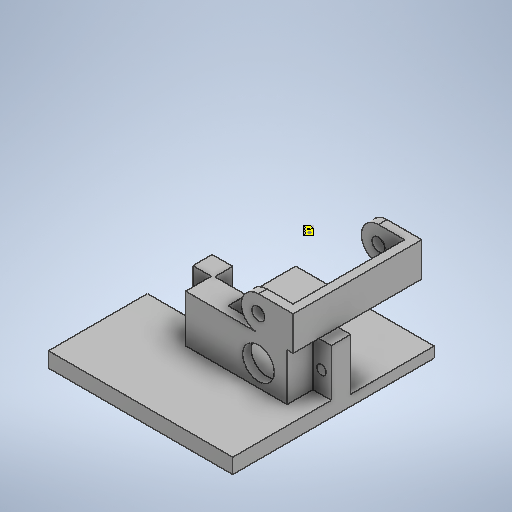
# Autodesk Inventor part: housing_shaft_link_base
Saved by Autodesk Inventor 2025 (Build 290162000, 162)
## iProperties
Created: 2025-09-17
Part Number: housing_shaft_link_base
Material: 一般
Document SubType Name: Modeling
Designer: sooo1
Density: 1 g/cm^3
Appearance: 滑らか - 標準の灰色
Author: sooo1
Autodesk Inventor part; units mm, degrees
sketch "スケッチ1" plane through (0, 0, 0) normal (0, 0, 1) x (1, 0, 0)
  circle A0 centre (0, 0) radius 1.5
  circle A1 centre (0, 0) radius 4
  line L0 (6.1, 4) -> (6.1, -4)
  line L1 (-27.76, 0) -> (17.46, 0) construction
  line L2 (6.1, 4) -> (0, 4)
  line L3 (6.1, -4) -> (0, -4)
  line L4 (6.1, -4) -> (8.1, -4)
  line L5 (8.1, -4) -> (8.1, 4)
  line L6 (8.1, 4) -> (6.1, 4)
  line L7 (0, -13.6) -> (0, 18.6) construction
  circle A2 centre (0, 10) radius 1.5
  circle A3 centre (0, 10) radius 4
  line L8 (6.1, 14) -> (6.1, 6)
  line L9 (6.1, 14) -> (0, 14)
  line L10 (6.1, 6) -> (0, 6)
  line L11 (6.1, 6) -> (8.1, 6)
  line L12 (8.1, 6) -> (8.1, 14)
  line L13 (8.1, 14) -> (6.1, 14)
  line L14 (-16.4, 6.05) -> (6.1, 6.05) construction
  line L15 (6.1, 6.05) -> (6.1, -6.05)
  line L16 (6.1, -6.05) -> (-16.4, -6.05) construction
  line L17 (-16.4, -6.05) -> (-16.4, 6.05)
  line L18 (-16.4, 6.05) -> (6.1, -6.05) construction
  line L19 (6.1, 6.05) -> (-16.4, -6.05) construction
  line L20 (-21.3, 6.05) -> (11, 6.05) construction
  line L21 (11, 6.05) -> (11, -6.05) construction
  line L22 (11, -6.05) -> (-21.3, -6.05)
  line L23 (-21.3, -6.05) -> (-21.3, 6.05) construction
  line L24 (-21.3, 6.05) -> (11, -6.05) construction
  line L25 (11, 6.05) -> (-21.3, -6.05) construction
  line L26 (-21.3, 0) -> (11, 0) construction
  circle A4 centre (-19, 0) radius 1.1
  line L27 (-5.15, 6.05) -> (-5.15, -6.05) construction
  circle A5 centre (0, 0) radius 2.425
  circle A6 centre (0, 0) radius 6.05
  circle A7 centre (0, 0) radius 9
  line L28 (8.1, -7) -> (-21.3, -7)
  line L29 (-21.3, -7) -> (-21.3, 6.05)
  line L30 (-21.3, 6.05) -> (8.1, 6.05)
  line L31 (8.1, 6.05) -> (8.1, -7)
  line L32 (-21.3, -5) -> (-20.943492, -5)
  line L33 (-20.943492, -5) -> (8.1, -5)
  circle A8 centre (8.7, 0) radius 1.1
  line L34 (8.1, 6.05) -> (11, 6.05)
  line L35 (11, 6.05) -> (11, -6.05)
  point P0 (6.1, 0)
  point P1 (6.1, 10)
  point P2 (-5.15, 0)
  point P3 (-5.15, 0)
  point P4 (-0.630476, 6.05)
  point P5 (8.1, 6.05)
  point P6 (8.1, -6.05)
  point P7 (0, 6.05)
  point P8 (-6.663145, 6.05)
  point P9 (-6.663145, -6.05)
  point P10 (0, -6.05)
  point P11 (6.1, 6.617401)
  point P12 (6.663145, 6.05)
  point P13 (0.630476, 6.05)
  point P14 (0.489992, 6.030125)
  point P15 (0.776209, 6)
  point P16 (8.062258, 4)
  point P17 (8.1, 3.923009)
  point P18 (8.062258, -4)
  point P19 (8.1, -3.923009)
  point P20 (6.708204, 6)
  dimension "d0" = 3
  dimension "d1" = 8
  dimension "d3" = 8
  dimension "d4" = 2
  dimension "d11" = 10
  dimension "d21" = 12.1
  dimension "d22" = 22.5
  dimension "d23" = 32.3
  dimension "d24" = 2.2
  dimension "d26" = 27.7
  dimension "d28" = 18
  dimension "d29" = 12.1
  dimension "d30" = 4.85
  dimension "d31" = 6.1
  dimension "d32" = 7
  dimension "d55" = 2
  constraints: 68 end point, 10 midpoint, 9 centre point, 7 collinear, 7 parallel, 6 coincident, 6 horizontal, 6 perpendicular, 5 point on line, 4 point on circle, 2 vertical, 1 concentric, 1 symmetric about line, 19 other
  measures "d0" diameter of A0
  measures "d1" diameter of A1
  measures "d3" distance of L0.start L0.end
  measures "d4" distance between parallel lines of L0 L5
  measures "d11" distance of point (0, 0) point (0, 10)
  measures "d21" distance of L14.end L15.end
  measures "d22" distance of L14.start L14.end
  measures "d23" distance of L20.start L20.end
  measures "d24" diameter of A4
  measures "d26" diameter of A4.centre L27
  measures "d28" diameter of A7
  measures "d29" diameter of A6
  measures "d30" diameter of A5
  measures "d31" distance from line of L15 A5.centre
  measures "d32" distance from line of L28 point (0, 0)
  measures "d55" distance between parallel lines of L28 L33
extrude "押し出し1" add sketch "スケッチ1" along normal blind 2 contours A1 | A1 L2 A6 L3 | L2 L0 L3 A6 | L6 A7 L5 A8 L4 L0 | L6 L5 A7 | A7 L5 L4 | L5 A8 | A5
extrude "押し出し2" add sketch "スケッチ1" against normal blind 7 contours L6 A7 L5 A8 L4 L0 | L6 L5 A7 | A7 L5 L4 | L5 A8
extrude "押し出し3" add sketch "スケッチ1" against normal blind 2 from surface at -7 contours A6 A3 L30 L8 L10 | L10 A3 A6 | L8 L30 A7 L11 | A3 A6 | A6 L30 A3 | A7 L30 L12 L11 | L30 A3 A7 L8 | L8 A7 L30 | A3 L30 A6 | L30 A3 A7 A2 | A7 L8 L13 L12 L30 | A7 A3 L9 L8 | A7 A2 A3
pattern_linear "矩形状パターン1" count 2 spacing 28 along (0, 0, -1) of "押し出し3"
ref_plane "作業平面1" through (0, 0, -17.5) normal (0, 0, 1) x (1, 0, 0)
extrude "押し出し4" add sketch "スケッチ1" against normal up to surface (10.5 mm away) from surface at -7 contours A0 | A1 | A1 L2 A6 L3 | A1 L3 A6 L33 A3 L10 L2 | A6 L10 L15 L2 | L2 L0 L3 A6 | L3 L15 L33 A6 | L6 A7 L5 A8 L4 L0 | L15 L11 A7 L6 | A6 A3 L30 L8 L10 | L10 A3 A6 | L4 A7 L33 L15 | L33 L15 L22 A6 | A6 L33 | A7 L11 L31 L6 | L6 L5 A7 | L8 L30 A7 L11 | A3 A6 | A6 L30 A3 | A7 L5 L4 | L4 L31 L33 A7 | L33 A7 L22 L15 | L22 A7 L28 | L22 A7 L33 A6 | L33 A7 L30 A3 A6 | A7 L30 L12 L11 | A3 L30 A6 | L33 L31 L22 A7 | A7 L28 L29 L22 | L22 L17 L33 A7 | L33 L17 L30 A7 | L5 A8 | L22 L31 L28 A7 | L22 L29 L32 L33 L17 | L33 L32 L29 L30 L17 | A4 | A5
ref_plane "作業平面2" through (0, 0, -13.3) normal (0, 0, 1) x (1, 0, 0)
extrude "押し出し6" cut sketch "スケッチ1" against normal blind 23.4 from surface at -13.3 contours A0 | A1 | A1 L2 A6 L3 | A1 L3 A6 L33 A3 L10 L2 | A6 L10 L15 L2 | L2 L0 L3 A6 | L3 L15 L33 A6 | A6 A3 L30 L8 L10 | L10 A3 A6 | L33 L15 L22 A6 | A6 L33 | A3 A6 | A6 L30 A3 | L22 A7 L33 A6 | L33 A7 L30 A3 A6 | A3 L30 A6 | L22 L17 L33 A7 | L33 L17 L30 A7 | A5
ref_plane "作業平面3" through (0, 0, -9) normal (0, 0, 1) x (1, 0, 0)
extrude "押し出し7" cut sketch "スケッチ1" against normal up to surface (4.3 mm away) from surface at -9 contours A0 | A1 | A1 L2 A6 L3 | A1 L3 A6 L33 A3 L10 L2 | L10 A3 A6 | A6 L33 | A3 A6 | L22 A7 L33 A6 | L33 A7 L30 A3 A6 | A3 L30 A6 | A5 picked at (-0.459231, 6.046871)
extrude "押し出し8" cut sketch "スケッチ1" against normal up to surface (9 mm away) contours A0 | A5
extrude "押し出し9" cut sketch "スケッチ1" against normal through all contours A4
extrude "押し出し10" add sketch "スケッチ1" against normal up to surface (28 mm away) from surface at -9 contours L22 A7 L28 | L8 A7 L30 | A7 L28 L29 L22 | A7 L8 L13 L12 L30 | L22 L31 L28 A7
extrude "押し出し11" cut sketch "スケッチ1" against normal up to surface (19.5 mm away) from surface at -17.5 contours A6 A3 L30 L8 L10 | L10 A3 A6 | L8 L30 A7 L11 | A3 A6 | A6 L30 A3 | A7 L30 L12 L11 | A3 L30 A6
sketch "スケッチ3" plane through (0, 4, 2) normal (0, 1, 0) x (1, 0, 0)
  line L0 (8.1, 0) -> (0, 0) projected
  line L1 (8.1, 9) -> (8.1, 0) projected
  line L2 (6.1, 9) -> (8.1, 9) projected
  line L3 (6.1, 2) -> (6.1, 9) projected
  line L4 (6.1, 2) -> (0, 2) projected
  line L5 (0, 2) -> (0, 0) projected
  line L6 (0, 2) -> (0, 2) projected
  line L7 (0, 2) -> (0, 0) projected
  line L8 (0, 0) -> (0, 0) projected
  line L9 (0, 2) -> (0, 0) projected
  line L10 (-4, 2) -> (-4, 0) projected
  line L11 (-4, 2) -> (0, 2) projected
  line L12 (-4, 0) -> (0, 0) projected
extrude "押し出し12" cut sketch "スケッチ3" against normal through all
extrude "押し出し13" add sketch "スケッチ1" along normal blind 10 and the other way blind 7 contours L33 L15 L22 A6 | A6 L33 | L33 A7 L22 L15 | L22 A7 L28 | L22 A7 L33 A6 | L33 L31 L22 A7 | A7 L28 L29 L22 | L22 L17 L33 A7 | L22 L31 L28 A7 | L22 L29 L32 L33 L17
sketch "スケッチ4" plane through (-21.3, 6.05, -17.5) normal (-1, 0, 0) x (0, 0, 1)
  line L0 (27.5, -13.05) -> (-19.5, -13.05) projected
  line L1 (27.5, -11.05) -> (27.5, -13.05) projected
  line L2 (10.5, -11.05) -> (27.5, -11.05) projected
  line L3 (10.5, 0) -> (10.5, -11.05) projected
  line L4 (10.5, 0) -> (0, 0) projected
  line L5 (0, -12.1) -> (0, 0) projected
  line L6 (0, -12.1) -> (-19.5, -12.1) projected
  line L7 (-19.5, -12.1) -> (-19.5, -13.05) projected
  line L8 (10.5, -11.05) -> (10.5, -13.05)
  point P0 (17.5, -6.05)
  constraints: 2 end point, 1 perpendicular, 1 point on line
extrude "押し出し14" add sketch "スケッチ4" along normal blind 10.7 contours L0 L8 L2 L1
sketch "スケッチ5" plane through (-21.3, -5, -47) normal (0, -1, 0) x (1, 0, 0)
  line L0 (29.4, 10) -> (29.4, 57) projected
  line L1 (29.4, 57) -> (-10.7, 57) projected
  line L2 (-10.7, 40) -> (-10.7, 57) projected
  line L3 (0, 40) -> (-10.7, 40) projected
  line L4 (0, 40) -> (0, 10) projected
  line L5 (0, 10) -> (29.4, 10) projected
  line L6 (-10.7, 43.5) -> (29.4, 43.5) construction
  line L7 (1.2, 51.1) -> (16.4, 51.1)
  line L8 (16.4, 51.1) -> (16.4, 35.9)
  line L9 (16.4, 35.9) -> (1.2, 35.9)
  line L10 (1.2, 35.9) -> (1.2, 51.1)
  line L11 (1.2, 51.1) -> (16.4, 35.9) construction
  line L12 (16.4, 51.1) -> (1.2, 35.9) construction
  line L13 (-10.7, 57) -> (-10.7, 40) projected
  line L14 (-10.7, 40) -> (-10.7, 33.9)
  line L15 (-10.7, 33.9) -> (0, 33.9)
  line L16 (29.4, 57) -> (-10.7, 57) projected
  point P0 (21.3, 47)
  point P1 (8.8, 43.5)
  dimension "d63" = 15.2
  dimension "d64" = 15.2
  dimension "d68" = 13.5
  dimension "d69" = 2
  dimension "d105" = 19.5
  constraints: 18 end point, 4 point on line, 3 perpendicular, 2 midpoint, 2 parallel, 1 horizontal, 1 vertical
  measures "d63" distance of L7.start L7.end
  measures "d64" distance of L9.end L7.start
  measures "d68" distance from line of point (8.8, 43.5) L1
  measures "d69" distance between parallel lines of L15 L9
  measures "d105" distance from line of L13 point (8.8, 43.5)
extrude "押し出し17" add sketch "スケッチ5" along normal blind 1.5 from surface at 2 contours L5 L4 L3 L2 L1 L0 | L7 L8 L9 L10
extrude "押し出し15" cut sketch "スケッチ5" against normal blind 2 from surface at 3.5 contours L7 L8 L9 L10
ref_plane "作業平面4" through (-12.5, -8.5, -11.1) normal (-1, 0, 0) x (0, 0, 1)
ref_plane "作業平面5" through (-20.1, -6.5, -3.5) normal (0, 0, 1) x (1, 0, 0)
extrude "押し出し16" add sketch "スケッチ5" along normal up to surface (3.5 mm away) contours L15 L14 L3 L4
extrude "押し出し18" add sketch "スケッチ1" against normal up to surface (10.5 mm away) from surface at -7 contours L6 A7 L5 A8 L4 L0 | L15 L11 A7 L6 | L4 A7 L33 L15 | A7 L11 L31 L6 | L4 L31 L33 A7 | L33 A7 L22 L15 | L31 L12 L34 L35 L22 L5 A7 A8 | A7 A8 L5 | A7 L30 L12 L11 | L33 L31 L22 A7 | L5 A8 A7 | A8 A7 L5 | L5 A8 | A8 A7
extrude "押し出し19" cut sketch "スケッチ1" against normal through all contours A8 A7 L5 | L5 A8 | A8 A7 picked at (8.4, 0)
sketch "スケッチ6" plane through (8.1, -5, 10) normal (1, 0, 0) x (0, 0, -1)
  line L0 (27.5, -1.05) -> (17, -1.05) projected
  line L1 (17, -1.05) -> (17, 0) projected
  line L2 (17, 0) -> (0, 0) projected
  line L3 (0, 0) -> (0, -3.5) projected
  line L4 (0, -3.5) -> (47, -3.5) projected
  line L5 (47, -1.05) -> (47, -3.5) projected
  line L6 (27.5, -1.05) -> (47, -1.05) projected
  point P0 (10, 5)
extrude "押し出し20" add sketch "スケッチ6" along normal up to surface (2.9 mm away)
sketch "スケッチ7" plane through (6.1, -6.05, -17.5) normal (0, 0, -1) x (-1, 0, 0)
  circle A0 centre (-2.6, 6.05) radius 1.1
  line L0 (-4.9, 0) -> (0, 0)
  line L1 (0, 0) -> (0, 12.1)
  line L2 (0, 12.1) -> (-2, 12.1)
  line L3 (-2, 12.1) -> (-4.9, 12.1)
  line L4 (-4.9, 12.1) -> (-4.9, 0)
  line L5 (0, 12.1) -> (0, 0)
  line L6 (0, 0) -> (6.1, 0)
  arc A1 (6.1, 12.1) -> (6.1, 0) centre (6.1, 6.05) ccw
  line L7 (0, 12.1) -> (6.1, 12.1)
  arc A2 (12.763145, 0) -> (12.763145, 12.1) centre (6.1, 6.05) ccw
  line L8 (12.763145, 0) -> (22.5, 0)
  line L9 (22.5, 0) -> (22.5, 12.1)
  line L10 (12.763145, 12.1) -> (22.5, 12.1)
  line L11 (22.5, 12.1) -> (22.5, 0)
  line L12 (22.5, 0) -> (27.4, 0)
  line L13 (27.4, 0) -> (27.4, 12.1)
  line L14 (27.4, 12.1) -> (22.5, 12.1)
  circle A3 centre (25.1, 6.05) radius 1.1
  line L15 (6.730476, 12.1) -> (12.763145, 12.1)
  line L16 (6.1, 0) -> (12.763145, 0)
  circle A4 centre (6.1, 6.05) radius 2.425
  line L17 (0, 12.1) -> (6.1, 12.1)
  line L18 (6.1, 12.1) -> (6.730476, 12.1)
  line L19 (-0.1, 12.1) -> (-0.1, 0)
  line L20 (-4.9, 0) -> (0, 0)
  line L21 (22.6, 12.1) -> (22.6, 0)
  line L22 (22.5, 0) -> (27.4, 0)
  arc A5 (6.1, 12.2) -> (6.1, -0.1) centre (6.1, 6.05) ccw
  arc A6 (12.83718, -0.067222) -> (12.83718, 12.167222) centre (6.1, 6.05) ccw
  circle A7 centre (6.1, 6.05) radius 3.7
  line L23 (15.2, 12.1) -> (15.2, 0)
  line L24 (27.4, 1.05) -> (-4.9, 1.05)
  line L25 (23.1, 1.05) -> (23.1, 12.1)
  line L26 (-0.6, 1.05) -> (-0.6, 12.1)
  line L27 (22.5, 12.1) -> (22.5, 0)
  line L28 (22.5, 0) -> (27.4, 0)
  line L29 (27.4, 0) -> (27.4, 12.1)
  line L30 (27.4, 12.1) -> (22.5, 12.1)
  point P0 (22.6, 0)
  point P1 (-0.1, 0)
  point P2 (12.89761, 0)
  point P3 (12.89761, 12.1)
  point P4 (4.995464, 12.1)
  point P5 (4.995464, 0)
  point P6 (15.2, 6.05)
  dimension "d80" = 0.1
  dimension "d81" = 0.1
  dimension "d84" = 0.1
  dimension "d85" = 0.1
  dimension "d99" = 2
  dimension "d101" = 2
  dimension "d104" = 7.4
  constraints: 12 end point, 10 point on line, 4 perpendicular, 4 point on circle, 3 centre point, 1 collinear, 1 tangent, 1 vertical
  measures "d80" distance between parallel lines of L19 L1
  measures "d81" distance between parallel lines of L9 L21
  measures "d84" radial gap between concentric circles of A1 A5
  measures "d85" radial gap between concentric circles of A2 A6
  measures "d99" distance from line of L25 A3.centre
  measures "d101" distance from line of L26 A0.centre
  measures "d104" diameter of A7
extrude "押し出し21" cut sketch "スケッチ7" against normal up to surface (4.2 mm away) contours L19 L24 L1 L0 | L19 L2 L1 A5 L24 | A5 L1 | L9 L24 L21 L12 | L9 L14 L21 L24
sketch "スケッチ7 outline for 押し出し22" plane through (6.1, -6.05, -17.5) normal (0, 0, -1) x (-1, 0, 0)
  arc A0 (12.763145, 12.1) -> (12.763145, 0) centre (6.1, 6.05) cw
  line L0 (12.763145, 0) -> (15.2, 0)
  line L1 (15.2, 0) -> (15.2, 12.1)
  line L2 (15.2, 12.1) -> (12.763145, 12.1)
  arc A1 (6.1, 0) -> (6.1, 12.1) centre (6.1, 6.05) cw
  line L3 (6.1, 12.1) -> (-0.1, 12.1)
  line L4 (-0.1, 12.1) -> (-0.1, 0)
  line L5 (-0.1, 0) -> (6.1, 0)
extrude "押し出し22" cut sketch "スケッチ7 outline for 押し出し22" against normal up to surface (8.5 mm away)
extrude "押し出し23" cut sketch "スケッチ7" against normal through all contours A7
extrude "押し出し26" cut sketch "スケッチ7" along normal blind 6 from surface at -10.5 contours L4 L3 L2 L26 L24 | L25 L14 L13 L24
